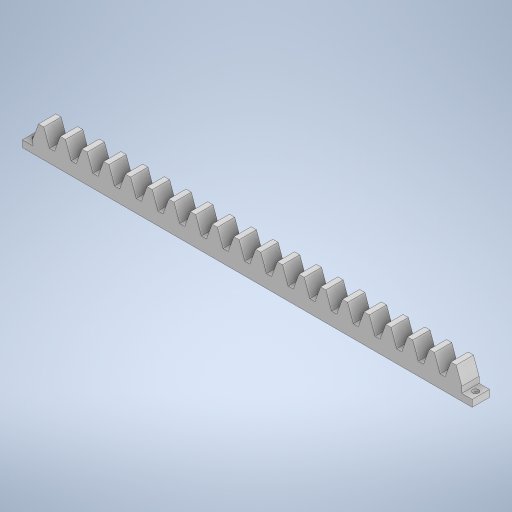
# Autodesk Inventor part: cremallera1
Saved by Autodesk Inventor 2023.2 (Build 272271030, 271C)
## iProperties
Created: 2023-03-04
Part Number: cremallera1
Material: Generic
Document SubType Name: Modeling
Designer: Cris Pat
Density: 1 g/cm^3
Appearance: Default
Author: Cris Pat
Autodesk Inventor part; units mm, degrees
ref_plane "YZ Plane" through (0, 0, 0) normal (1, 0, 0) x (0, 1, 0)
ref_plane "XZ Plane" through (0, 0, 0) normal (0, 1, 0) x (-1, 0, 0)
ref_plane "XY Plane" through (0, 0, 0) normal (0, 0, 1) x (1, 0, 0)
sketch "Sketch1" plane through (0, 0, 0) normal (0, 0, 1) x (1, 0, 0)
  line L0 (-8.1893, 41.3629) -> (-15.8199, 41.3629)
  line L1 (-8.1893, 41.3629) -> (0, 18.8629)
  line L2 (-8.1893, 41.3629) -> (26.4246, 41.3629) construction
  line L3 (-4.5496, 31.3629) -> (-19.4596, 31.3629) construction
  line L4 (-12.0046, 31.3629) -> (-12.0046, 41.3629) construction
  line L5 (-15.8199, 41.3629) -> (-24.0093, 18.8629)
  line L6 (-39.5993, 41.3629) -> (-47.2299, 41.3629)
  line L7 (-39.5993, 41.3629) -> (-31.41, 18.8629)
  line L8 (-39.5993, 41.3629) -> (-4.9854, 41.3629) construction
  line L9 (-35.9596, 31.3629) -> (-50.8696, 31.3629) construction
  line L10 (-43.4146, 31.3629) -> (-43.4146, 41.3629) construction
  line L11 (-47.2299, 41.3629) -> (-55.4193, 18.8629)
  line L12 (-71.0093, 41.3629) -> (-78.6399, 41.3629)
  line L13 (-71.0093, 41.3629) -> (-62.82, 18.8629)
  line L14 (-71.0093, 41.3629) -> (-36.3954, 41.3629) construction
  line L15 (-67.3696, 31.3629) -> (-82.2796, 31.3629) construction
  line L16 (-74.8246, 31.3629) -> (-74.8246, 41.3629) construction
  line L17 (-78.6399, 41.3629) -> (-86.8293, 18.8629)
  line L18 (-102.4193, 41.3629) -> (-110.0499, 41.3629)
  line L19 (-102.4193, 41.3629) -> (-94.23, 18.8629)
  line L20 (-102.4193, 41.3629) -> (-67.8054, 41.3629) construction
  line L21 (-98.7796, 31.3629) -> (-113.6896, 31.3629) construction
  line L22 (-106.2346, 31.3629) -> (-106.2346, 41.3629) construction
  line L23 (-110.0499, 41.3629) -> (-118.2393, 18.8629)
  line L24 (-133.8293, 41.3629) -> (-141.4599, 41.3629)
  line L25 (-133.8293, 41.3629) -> (-125.64, 18.8629)
  line L26 (-133.8293, 41.3629) -> (-99.2154, 41.3629) construction
  line L27 (-130.1896, 31.3629) -> (-145.0996, 31.3629) construction
  line L28 (-137.6446, 31.3629) -> (-137.6446, 41.3629) construction
  line L29 (-141.4599, 41.3629) -> (-149.6493, 18.8629)
  line L30 (-165.2393, 41.3629) -> (-172.8699, 41.3629)
  line L31 (-165.2393, 41.3629) -> (-157.05, 18.8629)
  line L32 (-165.2393, 41.3629) -> (-130.6254, 41.3629) construction
  line L33 (-161.5996, 31.3629) -> (-176.5096, 31.3629) construction
  line L34 (-169.0546, 31.3629) -> (-169.0546, 41.3629) construction
  line L35 (-172.8699, 41.3629) -> (-181.0593, 18.8629)
  line L36 (-196.6493, 41.3629) -> (-204.2799, 41.3629)
  line L37 (-196.6493, 41.3629) -> (-188.46, 18.8629)
  line L38 (-196.6493, 41.3629) -> (-162.0354, 41.3629) construction
  line L39 (-193.0096, 31.3629) -> (-207.9196, 31.3629) construction
  line L40 (-200.4646, 31.3629) -> (-200.4646, 41.3629) construction
  line L41 (-204.2799, 41.3629) -> (-212.4693, 18.8629)
  line L42 (-228.0593, 41.3629) -> (-235.6899, 41.3629)
  line L43 (-228.0593, 41.3629) -> (-219.87, 18.8629)
  line L44 (-228.0593, 41.3629) -> (-193.4454, 41.3629) construction
  line L45 (-224.4196, 31.3629) -> (-239.3296, 31.3629) construction
  line L46 (-231.8746, 31.3629) -> (-231.8746, 41.3629) construction
  line L47 (-235.6899, 41.3629) -> (-243.8793, 18.8629)
  line L48 (-259.4693, 41.3629) -> (-267.0999, 41.3629)
  line L49 (-259.4693, 41.3629) -> (-251.28, 18.8629)
  line L50 (-259.4693, 41.3629) -> (-224.8554, 41.3629) construction
  line L51 (-255.8296, 31.3629) -> (-270.7396, 31.3629) construction
  line L52 (-263.2846, 31.3629) -> (-263.2846, 41.3629) construction
  line L53 (-267.0999, 41.3629) -> (-275.2893, 18.8629)
  line L54 (-290.8793, 41.3629) -> (-298.5099, 41.3629)
  line L55 (-290.8793, 41.3629) -> (-282.69, 18.8629)
  line L56 (-290.8793, 41.3629) -> (-256.2654, 41.3629) construction
  line L57 (-287.2396, 31.3629) -> (-302.1496, 31.3629) construction
  line L58 (-294.6946, 31.3629) -> (-294.6946, 41.3629) construction
  line L59 (-298.5099, 41.3629) -> (-306.6993, 18.8629)
  line L60 (-322.2893, 41.3629) -> (-329.9199, 41.3629)
  line L61 (-322.2893, 41.3629) -> (-314.1, 18.8629)
  line L62 (-322.2893, 41.3629) -> (-287.6754, 41.3629) construction
  line L63 (-318.6496, 31.3629) -> (-333.5596, 31.3629) construction
  line L64 (-326.1046, 31.3629) -> (-326.1046, 41.3629) construction
  line L65 (-329.9199, 41.3629) -> (-338.1093, 18.8629)
  line L66 (-353.6993, 41.3629) -> (-361.3299, 41.3629)
  line L67 (-353.6993, 41.3629) -> (-345.51, 18.8629)
  line L68 (-353.6993, 41.3629) -> (-319.0854, 41.3629) construction
  line L69 (-350.0596, 31.3629) -> (-364.9696, 31.3629) construction
  line L70 (-357.5146, 31.3629) -> (-357.5146, 41.3629) construction
  line L71 (-361.3299, 41.3629) -> (-369.5193, 18.8629)
  line L72 (-385.1093, 41.3629) -> (-392.7399, 41.3629)
  line L73 (-385.1093, 41.3629) -> (-376.92, 18.8629)
  line L74 (-385.1093, 41.3629) -> (-350.4954, 41.3629) construction
  line L75 (-381.4696, 31.3629) -> (-396.3796, 31.3629) construction
  line L76 (-388.9246, 31.3629) -> (-388.9246, 41.3629) construction
  line L77 (-392.7399, 41.3629) -> (-400.9293, 18.8629)
  line L78 (-416.5193, 41.3629) -> (-424.1499, 41.3629)
  line L79 (-416.5193, 41.3629) -> (-408.33, 18.8629)
  line L80 (-416.5193, 41.3629) -> (-381.9054, 41.3629) construction
  line L81 (-412.8796, 31.3629) -> (-427.7896, 31.3629) construction
  line L82 (-420.3346, 31.3629) -> (-420.3346, 41.3629) construction
  line L83 (-424.1499, 41.3629) -> (-432.3393, 18.8629)
  line L84 (-447.9293, 41.3629) -> (-455.5599, 41.3629)
  line L85 (-447.9293, 41.3629) -> (-439.74, 18.8629)
  line L86 (-447.9293, 41.3629) -> (-413.3154, 41.3629) construction
  line L87 (-444.2896, 31.3629) -> (-459.1996, 31.3629) construction
  line L88 (-451.7446, 31.3629) -> (-451.7446, 41.3629) construction
  line L89 (-455.5599, 41.3629) -> (-463.7493, 18.8629)
  line L90 (-479.3393, 41.3629) -> (-486.9699, 41.3629)
  line L91 (-479.3393, 41.3629) -> (-471.15, 18.8629)
  line L92 (-479.3393, 41.3629) -> (-444.7254, 41.3629) construction
  line L93 (-475.6996, 31.3629) -> (-490.6096, 31.3629) construction
  line L94 (-483.1546, 31.3629) -> (-483.1546, 41.3629) construction
  line L95 (-486.9699, 41.3629) -> (-495.1593, 18.8629)
  line L96 (-510.7493, 41.3629) -> (-518.3799, 41.3629)
  line L97 (-510.7493, 41.3629) -> (-502.56, 18.8629)
  line L98 (-510.7493, 41.3629) -> (-476.1354, 41.3629) construction
  line L99 (-507.1096, 31.3629) -> (-522.0196, 31.3629) construction
  line L100 (-514.5646, 31.3629) -> (-514.5646, 41.3629) construction
  line L101 (-518.3799, 41.3629) -> (-526.5693, 18.8629)
  line L102 (-542.1593, 41.3629) -> (-549.7899, 41.3629)
  line L103 (-542.1593, 41.3629) -> (-533.97, 18.8629)
  line L104 (-542.1593, 41.3629) -> (-507.5454, 41.3629) construction
  line L105 (-538.5196, 31.3629) -> (-553.4296, 31.3629) construction
  line L106 (-545.9746, 31.3629) -> (-545.9746, 41.3629) construction
  line L107 (-549.7899, 41.3629) -> (-557.9793, 18.8629)
  line L108 (-573.5693, 41.3629) -> (-581.1999, 41.3629)
  line L109 (-573.5693, 41.3629) -> (-565.38, 18.8629)
  line L110 (-573.5693, 41.3629) -> (-538.9554, 41.3629) construction
  line L111 (-569.9296, 31.3629) -> (-584.8396, 31.3629) construction
  line L112 (-577.3846, 31.3629) -> (-577.3846, 41.3629) construction
  line L113 (-581.1999, 41.3629) -> (-589.3893, 18.8629)
  line L114 (-604.9793, 41.3629) -> (-612.6099, 41.3629)
  line L115 (-604.9793, 41.3629) -> (-596.79, 18.8629)
  line L116 (-604.9793, 41.3629) -> (-570.3654, 41.3629) construction
  line L117 (-601.3396, 31.3629) -> (-616.2496, 31.3629) construction
  line L118 (-608.7946, 31.3629) -> (-608.7946, 41.3629) construction
  line L119 (-612.6099, 41.3629) -> (-620.7993, 18.8629)
  line L120 (-620.7993, 18.8629) -> (-620.7993, 0)
  line L121 (-620.7993, 0) -> (0, 0)
  line L122 (0, 0) -> (0, 18.8629)
  line L123 (-24.0093, 18.8629) -> (-31.41, 18.8629)
  line L124 (-55.4193, 18.8629) -> (-62.82, 18.8629)
  line L125 (-86.8293, 18.8629) -> (-94.23, 18.8629)
  line L126 (-118.2393, 18.8629) -> (-125.64, 18.8629)
  line L127 (-149.6493, 18.8629) -> (-157.05, 18.8629)
  line L128 (-181.0593, 18.8629) -> (-188.46, 18.8629)
  line L129 (-212.4693, 18.8629) -> (-219.87, 18.8629)
  line L130 (-243.8793, 18.8629) -> (-251.28, 18.8629)
  line L131 (-275.2893, 18.8629) -> (-282.69, 18.8629)
  line L132 (-306.6993, 18.8629) -> (-314.1, 18.8629)
  line L133 (-338.1093, 18.8629) -> (-345.51, 18.8629)
  line L134 (-369.5193, 18.8629) -> (-376.92, 18.8629)
  line L135 (-400.9293, 18.8629) -> (-408.33, 18.8629)
  line L136 (-432.3393, 18.8629) -> (-439.74, 18.8629)
  line L137 (-463.7493, 18.8629) -> (-471.15, 18.8629)
  line L138 (-495.1593, 18.8629) -> (-502.56, 18.8629)
  line L139 (-526.5693, 18.8629) -> (-533.97, 18.8629)
  line L140 (-557.9793, 18.8629) -> (-565.38, 18.8629)
  line L141 (-589.3893, 18.8629) -> (-596.79, 18.8629)
  point P0 (2.0713, 13.1721)
  point P1 (-26.0805, 13.1721)
  point P2 (-29.3387, 13.1721)
  point P3 (-57.4905, 13.1721)
  point P4 (-60.7487, 13.1721)
  point P5 (-88.9005, 13.1721)
  point P6 (-92.1587, 13.1721)
  point P7 (-120.3105, 13.1721)
  point P8 (-123.5687, 13.1721)
  point P9 (-151.7205, 13.1721)
  point P10 (-154.9787, 13.1721)
  point P11 (-183.1305, 13.1721)
  point P12 (-186.3887, 13.1721)
  point P13 (-214.5405, 13.1721)
  point P14 (-217.7987, 13.1721)
  point P15 (-245.9505, 13.1721)
  point P16 (-249.2087, 13.1721)
  point P17 (-277.3605, 13.1721)
  point P18 (-280.6187, 13.1721)
  point P19 (-308.7705, 13.1721)
  point P20 (-312.0287, 13.1721)
  point P21 (-340.1805, 13.1721)
  point P22 (-343.4387, 13.1721)
  point P23 (-371.5905, 13.1721)
  point P24 (-374.8487, 13.1721)
  point P25 (-403.0005, 13.1721)
  point P26 (-406.2587, 13.1721)
  point P27 (-434.4105, 13.1721)
  point P28 (-437.6687, 13.1721)
  point P29 (-465.8205, 13.1721)
  point P30 (-469.0787, 13.1721)
  point P31 (-497.2305, 13.1721)
  point P32 (-500.4887, 13.1721)
  point P33 (-528.6405, 13.1721)
  point P34 (-531.8987, 13.1721)
  point P35 (-560.0505, 13.1721)
  point P36 (-563.3087, 13.1721)
  point P37 (-591.4605, 13.1721)
  point P38 (-594.7187, 13.1721)
  point P39 (-622.8705, 13.1721)
  point P40 (-59.1196, 18.8629)
  point P41 (0, 9.4315)
  dimension "d3" = 30
  dimension "d4" = 70
  dimension "d5" = 14.91
  dimension "d8" = 31.41
  dimension "d14" = 620.7993
  dimension "d15" = 18.8629
  dimension "d16" = 18.8629
  dimension "d18" = 13.1722
  dimension "d19" = 13.1722
  dimension "d20" = 24.0093
  dimension "d21" = 22.5
  dimension "d22" = 23.944
  dimension "d23" = 3.0107
  dimension "d24" = 18.8629
  constraints: 284 end point, 23 midpoint, 21 horizontal, 20 parallel, 20 perpendicular, 20 point on line, 2 symmetric about line, 1 coincident, 1 collinear, 1 vertical alignment, 322 other
  measures "d3" distance of L0.start point (2.071, 13.172)
  measures "d4" angle of L1 L2
  measures "d5" distance of L3.start L3.end
  measures "d8" distance of L0.start L6.start
  measures "d14" distance between parallel lines of L122 L120
  measures "d15" distance between parallel lines of L121 L123
  measures "d16" distance from line of L121 point (-59.12, 18.863)
  measures "d18" distance from line of L121 point (-88.901, 13.172)
  measures "d19" distance from line of L121 point (-29.339, 13.172)
  measures "d20" distance of L1.end L5.end
  measures "d21" vertical distance of L0.start L1.end
  measures "d22" distance of L0.end L5.end
  measures "d23" distance from line of L1 L8.end
  measures "d24" distance from line of L121 L120.start
extrude "Extrusion1" add sketch "Sketch1" along normal mid plane 25
sketch "Sketch2" plane through (0, 0, 0) normal (0, 1, 0) x (-1, 0, 0)
  line L0 (8.1893, -12.5) -> (8.1893, 12.5) construction
  line L1 (0, 12.5) -> (8.1893, 12.5) construction
  line L2 (0, -12.5) -> (0, 12.5) construction
  line L3 (8.1893, -12.5) -> (0, -12.5) construction
  line L4 (0, -12.5) -> (-15, -12.5)
  line L5 (-15, -12.5) -> (-15, 12.5)
  line L6 (-15, 12.5) -> (0, 12.5)
  line L7 (0, 12.5) -> (0, -12.5)
  line L8 (620.7993, -12.5) -> (620.7993, 12.5) construction
  line L9 (612.6099, 12.5) -> (620.7993, 12.5) construction
  line L10 (612.6099, 12.5) -> (612.6099, -12.5) construction
  line L11 (620.7993, -12.5) -> (612.6099, -12.5) construction
  line L12 (620.7993, -12.5) -> (635.7993, -12.5)
  line L13 (635.7993, -12.5) -> (635.7993, 12.5)
  line L14 (635.7993, 12.5) -> (620.7993, 12.5)
  line L15 (620.7993, 12.5) -> (620.7993, -12.5)
  point P0 (0, 0)
  dimension "d27" = 15
  dimension "d28" = 25
  dimension "d29" = 15
  dimension "d30" = 25
  constraints: 16 end point, 4 parallel, 2 horizontal, 2 perpendicular
  measures "d27" distance of L5.end L6.end
  measures "d28" distance between parallel lines of L4 L6
  measures "d29" distance of L14.end L13.end
  measures "d30" distance of L13.end L12.end
extrude "Extrusion2" add sketch "Sketch2" along normal blind 10
sketch "Sketch3" plane through (0, 10, 0) normal (0, 1, 0) x (1, 0, 0)
  line L0 (0, -12.5) -> (15, -12.5) construction
  line L1 (15, -12.5) -> (15, 12.5) construction
  line L2 (15, 12.5) -> (0, 12.5) construction
  line L3 (0, -12.5) -> (0, 12.5) construction
  line L4 (-635.7993, 12.5) -> (-635.7993, -12.5) construction
  line L5 (-635.7993, -12.5) -> (-620.7993, -12.5) construction
  line L6 (-620.7993, 12.5) -> (-620.7993, -12.5) construction
  line L7 (-620.7993, 12.5) -> (-635.7993, 12.5) construction
  line L8 (15, 12.5) -> (-635.7993, 12.5) construction
  line L9 (-635.7993, -12.5) -> (15, -12.5) construction
  line L10 (-310.3996, -12.5) -> (-310.3996, 12.5) construction
  circle A0 centre (7.5, 0) radius 2.65
  circle A1 centre (-628.2993, 0) radius 2.65
  point P0 (0, 0)
  point P1 (0, 0)
  point P2 (7.5, 12.5)
  dimension "d33" = 5.3
  constraints: 4 midpoint, 2 centre point, 2 end point, 1 horizontal alignment, 1 symmetric about line, 1 vertical alignment, 1 other
  measures "d33" diameter of A0
extrude "Extrusion3" cut sketch "Sketch3" against normal through all
sketch "Sketch4" plane through (0, 10, 0) normal (0, 1, 0) x (1, 0, 0)
  circle A0 centre (-628.2993, 0) radius 2.65 construction
  line L0 (-635.7993, 12.5) -> (-635.7993, -12.5) construction
  line L1 (-635.7993, -12.5) -> (-620.7993, -12.5) construction
  line L2 (-620.7993, 12.5) -> (-620.7993, -12.5) construction
  line L3 (-620.7993, 12.5) -> (-635.7993, 12.5) construction
  circle A1 centre (7.5, 0) radius 2.65 construction
  line L4 (0, -12.5) -> (15, -12.5) construction
  line L5 (15, -12.5) -> (15, 12.5) construction
  line L6 (15, 12.5) -> (0, 12.5) construction
  line L7 (0, -12.5) -> (0, 12.5) construction
  line L8 (15, 12.5) -> (-635.7993, 12.5) construction
  line L9 (-635.7993, -12.5) -> (15, -12.5) construction
  line L10 (-310.3996, 12.5) -> (-310.3996, -12.5) construction
  circle A2 centre (7.5, 0) radius 4.35
  circle A3 centre (-628.2993, 0) radius 4.35
  point P0 (0, 0)
  dimension "d36" = 8.7
  constraints: 2 centre point, 2 end point, 2 midpoint, 1 coincident, 1 symmetric about line, 1 other
  measures "d36" diameter of A2
extrude "Extrusion4" cut sketch "Sketch4" against normal blind 3.5
body "Solid1"
